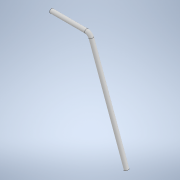
# Autodesk Inventor part: loganWalkerHandlePart
Saved by Autodesk Inventor 2022 (Build 260153070, 153G)
## iProperties
Created: 2021-06-06
Part Number: loganWalkerHandlePart
Material: Generic
Document SubType Name: Modeling
Designer: robst
Density: 1 g/cm^3
Appearance: Default
Author: robst
Autodesk Inventor part; units mm, degrees
ref_plane "YZ Plane" through (0, 0, 0) normal (1, 0, 0) x (0, 1, 0)
ref_plane "XZ Plane" through (0, 0, 0) normal (0, 1, 0) x (-1, 0, 0)
ref_plane "XY Plane" through (0, 0, 0) normal (0, 0, 1) x (1, 0, 0)
sketch "Sketch3" plane through (0, 0, 0) normal (0, 0, 1) x (1, 0, 0)
  line L0 (0, 508) -> (177.8, 508)
  line L1 (201.6601, 491.3095) -> (381, 0)
  arc A0 (201.6601, 491.3095) -> (177.8, 508) centre (177.8, 482.6) ccw
  line L2 (0, 0) -> (0, 508) construction
  dimension "d4" = 508
  dimension "d5" = 0
  dimension "d9" = 25.4
  dimension "d10" = 177.8
  dimension "d13" = 381
  constraints: 6 end point, 2 point on circle, 2 tangent, 1 centre point, 1 horizontal, 1 vertical
  measures "d4" distance from line of L0 L2.start
  measures "d5" vertical distance of L1.end L2.start
  measures "d9" radius of A0
  measures "d10" distance of L0.end L0.start
  measures "d13" distance of L1.end L2.start
sketch "Sketch4" plane through (0, 0, 0) normal (1, 0, 0) x (0, 1, 0)
  circle A0 centre (508, 0) radius 10.16
  point P0 (0, 0)
  dimension "d7" = 20.32
  dimension "d8" = 508
  constraints: 1 centre point
  measures "d7" diameter of A0
  measures "d8" distance of point (0, 0) A0.centre
sweep "Sweep1" add profiles "Sketch4" path "Sketch3"
equation "\"d4\" = handleHeight"
equation "\"d9\" = handleRadius"
equation "\"d10\" = handleLength"
equation "\"d13\" = handleBottomLength"
equation "\"d7\" = tubingOutsideDiameter"
equation "\"d8\" = handleHeight"
equation "\"handleHeight\" = 508"
equation "\"handleLength\" = 177.8"
equation "\"tubingOutsideDiameter\" = 20.32"
equation "\"handleRadius\" = 25.4"
equation "\"handleBottomLength\" = 381"
body "Solid1"
